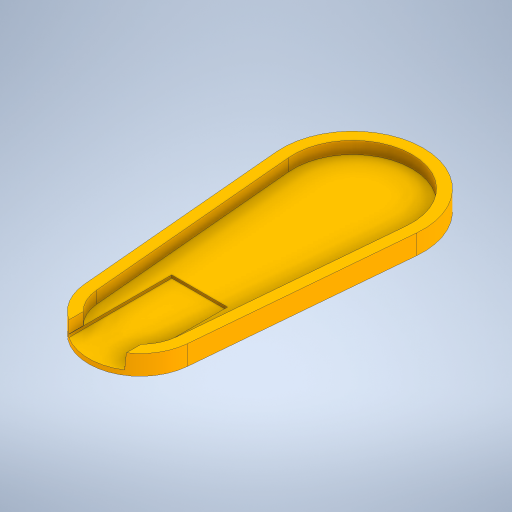
# Autodesk Inventor part: Tapa1
Saved by Autodesk Inventor 2024 (Build 280153000, 153)
## iProperties
Created: 2024-04-28
Part Number: Tapa1
Material: Generic
Document SubType Name: Modeling
Designer: samue
Density: 1 g/cm^3
Appearance: Default
Author: samue
## iProperties of the stored document Tapa1_3DPrint.ipt
Created: 2024-04-28
Part Number: Tapa1_3DPrint
Material: Generic
Document SubType Name: Modeling
Designer: samue
Density: 1 g/cm^3
Appearance: Default
Author: samue
Autodesk Inventor part; units mm, degrees
ref_plane "YZ Plane" through (0, 0, 0) normal (1, 0, 0) x (0, 1, 0)
ref_plane "XZ Plane" through (0, 0, 0) normal (0, 1, 0) x (-1, 0, 0)
ref_plane "XY Plane" through (0, 0, 0) normal (0, 0, 1) x (1, 0, 0)
sketch "Sketch1" plane through (0, 0, 0) normal (0, 1, 0) x (-1, 0, 0)
  arc A0 (5.4799, 0.7804) -> (-5.4769, 0.7804) centre (0.0015, 0.2935) ccw
  arc A1 (-7.4691, -21.6354) -> (7.472, -21.6354) centre (0.0015, -22.2993) ccw
  line L0 (-5.4769, 0.7804) -> (-7.4691, -21.6354)
  line L1 (5.4799, 0.7804) -> (7.472, -21.6354)
  line L2 (6.2767, -21.7416) -> (4.2846, 0.6742)
  arc A2 (4.2846, 0.6742) -> (-4.2816, 0.6742) centre (0.0015, 0.2935) ccw
  line L3 (-4.2816, 0.6742) -> (-6.2738, -21.7416)
  arc A3 (-6.2738, -21.7416) -> (6.2767, -21.7416) centre (0.0015, -22.2993) ccw
  dimension "d18" = 11
  dimension "d19" = 15
  dimension "d22" = 1.2
  constraints: 8 end point, 8 point on circle, 4 centre point, 4 tangent, 1 vertical alignment, 3 other
  measures "d18" diameter of A0
  measures "d19" diameter of A1
  measures "d22" distance between parallel lines of L1 L2
extrude "Extrusion7" add sketch "Sketch1" along normal blind 2.1
extrude "Extrusion8" add sketch "Sketch1" along normal blind 0.8 contours A3 L3 A2 L2
sketch "Sketch5" plane through (0, 0, 0) normal (0, 0, 1) x (1, 0, 0)
  line L0 (-3.019, 0.8) -> (2.981, 0.8)
  line L1 (5.4769, 0) -> (-5.4799, 0) projected
  line L2 (-3.019, 0.8) -> (-3.019, 4.3274)
  line L3 (-3.019, 4.3274) -> (3.2255, 4.3274)
  line L4 (3.2255, 4.3274) -> (2.981, 0.8)
  point P0 (0, 0)
  point P1 (-0.0015, 0)
  dimension "d27" = 6
  dimension "d28" = 0.8
  constraints: 8 end point, 1 horizontal, 1 midpoint, 1 vertical
  measures "d27" distance of L0.start L0.end
  measures "d28" distance from line of L0 point (-0.001, 0)
extrude "Extrusion9" cut sketch "Sketch5" along normal blind 14.7
sketch "Sketch6" plane through (0, 0.8, 0) normal (0, 1, 0) x (1, 0, 0)
  line L0 (-2.99, -5.9206) -> (2.938, -5.9206)
  line L1 (2.938, -5.9206) -> (2.938, 6.0287)
  line L2 (2.938, 6.0287) -> (-2.99, 6.0287)
  line L3 (-2.99, 6.0287) -> (-2.99, -5.9206)
  point P0 (0, 0)
  constraints: 8 end point, 2 parallel, 1 horizontal, 1 perpendicular
extrude "Extrusion10" cut sketch "Sketch6" against normal blind 0.3
body "Solid4"
